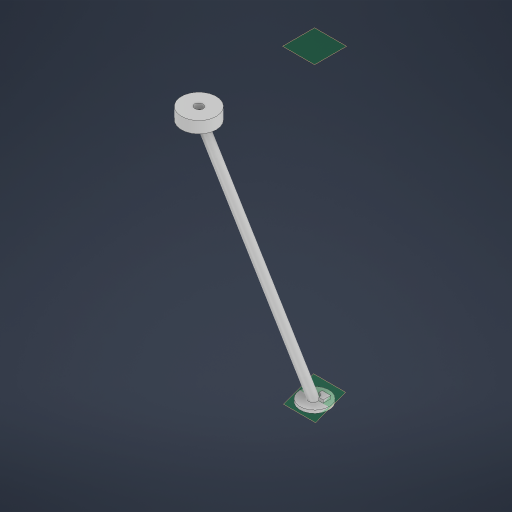
# Autodesk Inventor part: Legs
Saved by Autodesk Inventor 2023.2 (Build 272271030, 271C)
## iProperties
Created: 2023-04-10
Part Number: Legs
Material: Aluminum 6061
Document SubType Name: Modeling
Designer: ckeer
Density: 2.7 g/cm^3
Appearance: Aluminum - Polished
Author: ckeer
Autodesk Inventor part; units mm, degrees
ref_plane "YZ Plane" through (0, 0, 0) normal (1, 0, 0) x (0, 1, 0)
ref_plane "XZ Plane" through (0, 0, 0) normal (0, 1, 0) x (-1, 0, 0)
ref_plane "XY Plane" through (0, 0, 0) normal (0, 0, 1) x (1, 0, 0)
sketch "Sketch1" plane through (0, 0, 0) normal (0, 1, 0) x (-1, 0, 0)
  circle A0 centre (0, 0) radius 63.5
  dimension "d0" = 127
  constraints: 1 centre point, 1 coincident
  measures "d0" diameter of A0
extrude "Extrusion1" add sketch "Sketch1" along normal blind 12.7
sketch "Sketch2" plane through (0, 12.7, 0) normal (0, 1, 0) x (1, 0, 0)
  circle A0 centre (0, 0) radius 19.05
  circle A1 centre (0, 0) radius 63.5
  line L0 (0, 0) -> (37.718266, 0)
  line L1 (37.718266, 0) -> (37.718266, 33.673151)
  line L2 (37.718266, 33.673151) -> (0, 33.673151)
  line L3 (0, 33.673151) -> (0, 0)
  point P0 (63.5, 0)
  point P1 (0, 19.05)
  point P2 (19.05, 0)
  dimension "d3" = 38.1
  constraints: 8 end point, 2 parallel, 1 centre point, 1 coincident, 1 horizontal, 1 horizontal alignment, 1 perpendicular, 1 other
  measures "d3" diameter of A0
extrude "Extrusion2" add sketch "Sketch2" along normal blind 12.7 contours A0 L3 L2 L1 L0
ref_plane "Work Plane1" through (9.525, 12.7, 0) normal (0, -0.9356646, -0.3528907) x (-1, 0, 0)
sketch "Sketch3" plane through (9.525, 12.7, 0) normal (0, -0.9356646, -0.3528907) x (-1, 0, 0)
  circle A0 centre (9.525, -4.481711) radius 19.05
  dimension "d6" = 38.1
  constraints: 1 centre point, 1 coincident
  measures "d6" diameter of A0
extrude "Extrusion3" add sketch "Sketch3" along normal blind 4.826
sketch "Sketch4" plane through (9.525, 12.7, 0) normal (0, 0.9356646, 0.3528907) x (1, 0, 0)
  circle A0 centre (-9.525, -4.481711) radius 19.05
  constraints: 1 centre point, 1 coincident
extrude "Extrusion4" add sketch "Sketch4" along normal blind 1422.4
ref_plane "Work Plane2" through (0, 1346.2, 0) normal (0, -1, 0) x (1, 0, 0)
sketch "Sketch5" plane through (0, 1346.2, 0) normal (0, -1, 0) x (1, 0, 0)
  ellipse E0 centre (0, 506.145041) end of major axis (19.05, 506.145041) minor radius 17.82441
  circle A0 centre (0, 506.145041) radius 76.2
  point P0 (0, 0)
  dimension "d12" = 152.4
  constraints: 1 centre point, 1 coincident
  measures "d12" diameter of A0
extrude "Extrusion5" add sketch "Sketch5" along normal blind 25.4 and the other way blind 25.4
body "Solid1"
